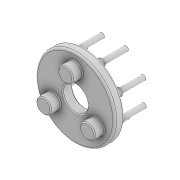
# Autodesk Inventor part: Connection disc of gear
Saved by Autodesk Inventor 2020.3 (Build 243373010, 373A)
## iProperties
Created: 2021-05-02
Part Number: Connection disc of gear
Material: Generic
Document SubType Name: Modeling
Designer: marti
Density: 1 g/cm^3
Appearance: Default
Author: marti
Autodesk Inventor part; units mm, degrees
ref_plane "YZ Plane" through (0, 0, 0) normal (1, 0, 0) x (0, 1, 0)
ref_plane "XZ Plane" through (0, 0, 0) normal (0, 1, 0) x (-1, 0, 0)
ref_plane "XY Plane" through (0, 0, 0) normal (0, 0, 1) x (1, 0, 0)
sketch "Sketch1" plane through (0, 0, 0) normal (0, 0, 1) x (1, 0, 0)
  circle A0 centre (-12.8375, 28.8334) radius 2.5
  circle A1 centre (11.3109, 29.4658) radius 2.5
  circle A2 centre (28.8334, 12.8375) radius 2.5
  circle A3 centre (29.4658, -11.3109) radius 2.5
  circle A4 centre (12.8375, -28.8334) radius 2.5
  circle A5 centre (-11.3109, -29.4658) radius 2.5
  circle A6 centre (-28.8334, -12.8375) radius 2.5
  circle A7 centre (-29.4658, 11.3109) radius 2.5
  circle A8 centre (0, 0) radius 31.5621
  circle A9 centre (0, 0) radius 40
  dimension "d0" = 80
  constraints: 9 centre point, 2 coincident, 3 other
  measures "d0" diameter of A9
extrude "Extrusion1" add sketch "Sketch1" against normal blind 30 contours A0 A8 | A8 A0 | A8 A1 | A1 A8 | A8 A7 | A7 A8 | A8 A2 | A2 A8 | A8 A6 | A6 A8 | A8 A5 | A5 A8 | A8 A3 | A3 A8 | A8 A4 | A4 A8
extrude "Extrusion2" add sketch "Sketch1" along normal blind 10 contours A0 A8 | A0 A8 A1 A2 A3 A4 A5 A6 A7 | A8 A0 | A8 A1 | A1 A8 | A8 A7 | A7 A8 | A8 A2 | A2 A8 | A8 A6 | A6 A8 | A8 A5 | A5 A8 | A8 A3 | A3 A8 | A8 A4 | A4 A8 | A9
sketch "Sketch2" plane through (0, 0, 0) normal (0, 0, -1) x (-1, 0, 0)
  point P0 (0, 0)
sketch "Sketch3" plane through (0, 0, 0) normal (0, 0, -1) x (-1, 0, 0)
  circle A0 centre (-11.3109, 29.4658) radius 2.5 projected
  circle A1 centre (-11.3109, 29.4658) radius 4
  point P0 (0, 0)
  dimension "d8" = 8
  constraints: 1 centre point, 1 coincident
  measures "d8" diameter of A1
extrude "Extrusion3" add sketch "Sketch3" along normal blind 5
pattern_circular "Circular Pattern1" count 8 over 360 about axis through (0, 0, -10) along (0, 0, 1) of "Extrusion3"
fillet "Fillet1" radius 2 1 edges at (-40, 0, 10)
fillet "Fillet2" radius 2 1 edges at (-40, 0, 0)
chamfer "Chamfer2" distance 0.5 angle 45 8 edges at (29.4658, -15.3109, 0) (31.6619, 10.0091, 0) (15.3109, 29.4658, 0) (-10.0091, 31.6619, 0) (-29.4658, 15.3109, 0) (10.0091, -31.6619, 0) (-15.3109, -29.4658, 0) (-31.6619, -10.0091, 0)
sketch "Sketch4" plane through (0, 0, 10) normal (0, 0, 1) x (1, 0, 0)
  circle A0 centre (0, 0) radius 12.5
  dimension "d19" = 25
  constraints: 1 centre point, 1 coincident
  measures "d19" diameter of A0
extrude "Extrusion4" cut sketch "Sketch4" against normal through all
sketch "Sketch5" plane through (0, 0, 10) normal (0, 0, 1) x (1, 0, 0)
  circle A0 centre (0, 25.5) radius 7.5
  circle A1 centre (0, 0) radius 12.5 projected
  circle A2 centre (0, 0) radius 38 projected
  dimension "d22" = 76
  dimension "d23" = 25
  dimension "d24" = 25.5
  dimension "d25" = 15
  constraints: 1 centre point
  measures "d22" diameter of A2
  measures "d23" diameter of A1
  measures "d24" distance of A0.centre point (0, 0)
  measures "d25" diameter of A0
extrude "Extrusion5" add sketch "Sketch5" along normal blind 10 contours A0
fillet "Fillet3" radius 1 1 edges at (-7.5, 25.5, 10)
chamfer "Chamfer3" distance 1 angle 45 1 edges at (-7.5, 25.5, 20)
pattern_circular "Circular Pattern2" count 3 over 360 about axis through (0, 0, -10) along (0, 0, 1) of "Extrusion5", "Fillet3", "Chamfer3"
chamfer "Chamfer4" distance 1 angle 45 2 edges at (-12.5, 0, 10) (-12.5, 0, 0)
body "Solid1"
